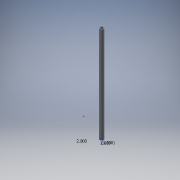
# Autodesk Inventor part: Gas Hose
Saved by Autodesk Inventor 2019 (Build 230136000, 136)
## iProperties
Created: 2019-11-15
Part Number: Gas Hose
Material: Generic
Document SubType Name: Modeling
Designer: Administrator
Density: 1 g/cm^3
Appearance: Default
Author: Administrator
Autodesk Inventor part; units mm, degrees
ref_plane "YZ Plane" through (0, 0, 0) normal (1, 0, 0) x (0, 1, 0)
ref_plane "XZ Plane" through (0, 0, 0) normal (0, 1, 0) x (-1, 0, 0)
ref_plane "XY Plane" through (0, 0, 0) normal (0, 0, 1) x (1, 0, 0)
sketch "Sketch2" plane through (0, 0, 0) normal (0, 1, 0) x (-1, 0, 0)
  circle A0 centre (0, 0) radius 19.05
  circle A1 centre (0, 0) radius 25.4
  dimension "d3" = 38.1
  dimension "d4" = 50.8
  constraints: 2 centre point, 2 coincident
  measures "d3" diameter of A0
  measures "d4" diameter of A1
sketch3d "3D Sketch1"
  line L0 (0, -266.153, -266.153) -> (0, 1003.847, -266.153)
  dimension "d1" = 1270
  dimension "d2" = 90
sweep "Sweep1" add profiles "Sketch2" path "3D Sketch1"
ref_plane "Work Plane2" through (-353.1457, -521.6169, -83.6447) normal (0.6592, 0, -0.752) x (0, -1, 0)
sketch "Sketch3" plane through (-353.1457, -521.6169, -83.6447) normal (0.6592, 0, -0.752) x (0, -1, 0)
  circle A0 centre (0, 0) radius 25.4
  point P0 (-521.6169, -320.7019)
  dimension "d7" = 50.8
  constraints: 1 centre point
  measures "d7" diameter of A0
sketch "Sketch4" plane through (0, -266.153, 0) normal (0, -1, 0) x (1, 0, 0)
  circle A0 centre (0, 0) radius 19.05 construction
  circle A1 centre (0, 0) radius 19.05
  circle A2 centre (0, 0) radius 25.4 construction
  point P0 (0, 0)
  dimension "d8" = 38.1
  dimension "d9" = 50.8
  constraints: 2 centre point, 2 coincident
  measures "d8" diameter of A0
  measures "d9" diameter of A2
body "Solid1"
